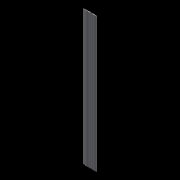
# Autodesk Inventor part: 3d_LM - Top Wire - Phantom
Saved by Autodesk Inventor 2018.3 (Build 223284000, 284)
## iProperties
Category: 0
Created: 2026-02-16
Part Number: 3d_LM - Top Wire - Phantom
Material: Genérico
Document SubType Name: Modeling
Designer: aca6
Density: 1 g/cm^3
Appearance: Valor por defecto
Manufacturer-1: {"Link": "", "Name": "\nEmbention Sistemas Inteligentes S.A.", "PartNumber": "3d_LM - Top Wire", "partner_id": false}
Manufacturer-2: {"Link": "", "Name": "", "PartNumber": "", "partner_id": false}
Manufacturer-3: {"Link": "", "Name": "", "PartNumber": "", "partner_id": false}
Manufacturer-4: {"Link": "", "Name": "", "PartNumber": "", "partner_id": false}
Manufacturer-5: {"Link": "", "Name": "", "PartNumber": "", "partner_id": false}
Provider-1: {"Link": "", "Name": "", "PartNumber": "", "partner_id": false}
Provider-2: {"Link": "", "Name": "", "PartNumber": "", "partner_id": false}
Provider-3: {"Link": "", "Name": "", "PartNumber": "", "partner_id": false}
Provider-4: {"Link": "", "Name": "", "PartNumber": "", "partner_id": false}
Provider-5: {"Link": "", "Name": "", "PartNumber": "", "partner_id": false}
odoo_id: 22904
odoo_internal_code: P015269
odoo_model: product.product
odoo_x2o_application_version: 12.0.4.20
odoo_d2o_version: 12.0.1.6.0
Author: aca6
Autodesk Inventor part; units mm, degrees
ref_plane "YZ Plane" through (0, 0, 0) normal (1, 0, 0) x (0, 1, 0)
ref_plane "XZ Plane" through (0, 0, 0) normal (0, 1, 0) x (-1, 0, 0)
sketch "Sketch1" plane through (0, 0, 0) normal (0, 0, 1) x (1, 0, 0)
  line L0 (21.5482, -2.9223) -> (19.9915, -2.9223) projected
  arc A0 (15.9111, -2.9223) -> (19.9915, -2.9223) centre (17.9513, -2.7223) ccw projected
  line L1 (15.9111, -2.9223) -> (15.4915, -2.9223) projected
  arc A1 (11.4111, -2.9223) -> (15.4915, -2.9223) centre (13.4513, -2.7223) ccw projected
  line L2 (11.4111, -2.9223) -> (10.9915, -2.9223) projected
  arc A2 (6.9111, -2.9223) -> (10.9915, -2.9223) centre (8.9513, -2.7223) ccw projected
  line L3 (6.9111, -2.9223) -> (5.3544, -2.9223) projected
  arc A3 (3.5482, -2.9223) -> (5.3544, -2.9223) centre (4.4513, -2.7223) ccw projected
  line L4 (3.5482, -2.9223) -> (1.9915, -2.9223) projected
  arc A4 (-2.0889, -2.9223) -> (1.9915, -2.9223) centre (-0.0487, -2.7223) ccw projected
  line L5 (-2.0889, -2.9223) -> (-2.5085, -2.9223) projected
  arc A5 (-6.5889, -2.9223) -> (-2.5085, -2.9223) centre (-4.5487, -2.7223) ccw projected
  line L6 (-6.5889, -2.9223) -> (-7.0085, -2.9223) projected
  arc A6 (-11.0889, -2.9223) -> (-7.0085, -2.9223) centre (-9.0487, -2.7223) ccw projected
  line L7 (-11.0889, -2.9223) -> (-11.5085, -2.9223) projected
  arc A7 (-15.5889, -2.9223) -> (-11.5085, -2.9223) centre (-13.5487, -2.7223) ccw projected
  line L8 (-15.5889, -2.9223) -> (-17.1712, -2.9223) projected
  arc A8 (-18.9262, -2.9223) -> (-17.1712, -2.9223) centre (-18.0487, -2.7223) ccw projected
  line L9 (-18.9262, -2.9223) -> (-21.6712, -2.9223) projected
  arc A9 (-23.4262, -2.9223) -> (-21.6712, -2.9223) centre (-22.5487, -2.7223) ccw projected
  line L10 (-23.4262, -2.9223) -> (-29.4262, -2.9223) projected
  line L11 (-29.4262, -2.9223) -> (-29.4262, -2.7223) projected
  line L12 (-29.4262, -2.7223) -> (-35.4262, -2.7223) projected
  line L13 (-35.4262, -2.7223) -> (-35.4262, -7.7223) projected
  line L14 (-35.4262, -7.7223) -> (35.3544, -7.7223) projected
  line L15 (35.3544, -7.7223) -> (35.3544, -2.7223) projected
  line L16 (35.3544, -2.7223) -> (29.3544, -2.7223) projected
  line L17 (29.3544, -2.7223) -> (29.3544, -2.9223) projected
  line L18 (29.3544, -2.9223) -> (23.3544, -2.9223) projected
  arc A10 (21.5482, -2.9223) -> (23.3544, -2.9223) centre (22.4513, -2.7223) ccw projected
  line L19 (19.9915, -2.5223) -> (21.5482, -2.5223) projected
  arc A11 (23.3544, -2.5223) -> (21.5482, -2.5223) centre (22.4513, -2.7223) ccw projected
  line L20 (23.3544, -2.5223) -> (29.3544, -2.5223) projected
  line L21 (29.3544, -2.5223) -> (29.3544, -2.7223) projected
  line L22 (29.3544, -2.7223) -> (35.3544, -2.7223) projected
  line L23 (35.3544, -2.7223) -> (35.3544, 2.2777) projected
  line L24 (35.3544, 2.2777) -> (-35.4262, 2.2777) projected
  line L25 (-35.4262, 2.2777) -> (-35.4262, -2.7223) projected
  line L26 (-35.4262, -2.7223) -> (-29.4262, -2.7223) projected
  line L27 (-29.4262, -2.7223) -> (-29.4262, -2.5223) projected
  line L28 (-29.4262, -2.5223) -> (-23.4262, -2.5223) projected
  arc A12 (-21.6712, -2.5223) -> (-23.4262, -2.5223) centre (-22.5487, -2.7223) ccw projected
  line L29 (-21.6712, -2.5223) -> (-18.9262, -2.5223) projected
  arc A13 (-17.1712, -2.5223) -> (-18.9262, -2.5223) centre (-18.0487, -2.7223) ccw projected
  line L30 (-17.1712, -2.5223) -> (-15.5889, -2.5223) projected
  arc A14 (-11.5085, -2.5223) -> (-15.5889, -2.5223) centre (-13.5487, -2.7223) ccw projected
  line L31 (-11.5085, -2.5223) -> (-11.0889, -2.5223) projected
  arc A15 (-7.0085, -2.5223) -> (-11.0889, -2.5223) centre (-9.0487, -2.7223) ccw projected
  line L32 (-7.0085, -2.5223) -> (-6.5889, -2.5223) projected
  arc A16 (-2.5085, -2.5223) -> (-6.5889, -2.5223) centre (-4.5487, -2.7223) ccw projected
  line L33 (-2.5085, -2.5223) -> (-2.0889, -2.5223) projected
  arc A17 (1.9915, -2.5223) -> (-2.0889, -2.5223) centre (-0.0487, -2.7223) ccw projected
  line L34 (1.9915, -2.5223) -> (3.5482, -2.5223) projected
  arc A18 (5.3544, -2.5223) -> (3.5482, -2.5223) centre (4.4513, -2.7223) ccw projected
  line L35 (5.3544, -2.5223) -> (6.9111, -2.5223) projected
  arc A19 (10.9915, -2.5223) -> (6.9111, -2.5223) centre (8.9513, -2.7223) ccw projected
  line L36 (10.9915, -2.5223) -> (11.4111, -2.5223) projected
  arc A20 (15.4915, -2.5223) -> (11.4111, -2.5223) centre (13.4513, -2.7223) ccw projected
  line L37 (15.4915, -2.5223) -> (15.9111, -2.5223) projected
  arc A21 (19.9915, -2.5223) -> (15.9111, -2.5223) centre (17.9513, -2.7223) ccw projected
  arc A22 (21.5482, -2.9223) -> (21.5482, -2.5223) centre (22.4513, -2.7223) ccw
  arc A23 (-21.6712, -2.5223) -> (-21.6712, -2.9223) centre (-22.5487, -2.7223) ccw
  point P0 (0, 0)
  constraints: 4 end point, 4 point on circle, 2 centre point, 2 coincident, 2 concentric
ref_plane "Work Plane1" through (-35.4262, -2.7223, -450) normal (0, 0, -1) x (0, 1, 0)
extrude "Extrusion1" add sketch "Sketch1" against normal up to surface (450 mm away) contours L0 A0 L1 A1 L2 A2 L3 A3 L4 A4 L5 A5 L6 A6 L7 A7 L8 A8 L9 A9 A23 A12 L29 A13 L30 A14 L31 A15 L32 A16 L33 A17 L34 A18 L35 A19 L36 A20 L37 A21 L19 A11 A22 A10
body "Solid1"
